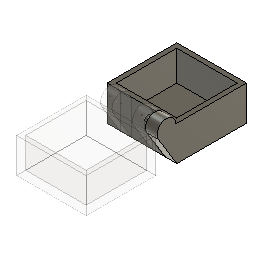
Day20BoxWithHinges (Autodesk Fusion 360 design; units mm, degrees)
part number: 2025-12-04-14-52-37-704
part number: 2025-12-04-18-52-37-317
part number: 2025-12-04-21-05-21-609
Autodesk Fusion 360 part; units mm, degrees
sketch "Sketch1" plane through (0, 0, 0) normal (0, 0, 1) x (1, 0, 0) in component "BoxBottom"
  line L0 (0, 0) -> (30, 0)
  line L1 (30, 0) -> (30, 30)
  line L2 (30, 30) -> (0, 30)
  line L3 (0, 30) -> (0, 0)
  dimension "d3" = 30
  dimension "d4" = 30
  constraint horizontal L0
  constraint vertical L1
  constraint horizontal L2
  constraint vertical L3
  constraint coincident L0.start L3.end
  measures "d3" distance of L0.start L2.end
  measures "d4" distance of L1.end L2.end
extrude "Extrude1" add sketch "Sketch1" along normal blind 15 makes body 1 in component "BoxBottom"
shell "Shell1" thickness 2 removed faces 1 at (10, 20, 15) on bodies 1 in component "BoxBottom"
sketch "Sketch1 (2)" plane through (0, 0, 0) normal (0, 0, 1) x (1, 0, 0) in component "BoxTop"
  line L0 (0, 0) -> (30, 0)
  line L1 (30, 0) -> (30, 30)
  line L2 (30, 30) -> (0, 30)
  line L3 (0, 30) -> (0, 0)
  dimension "d3_1" = 30
  dimension "d4_1" = 30
  constraint horizontal L0
  constraint vertical L1
  constraint horizontal L2
  constraint vertical L3
  constraint coincident L0.start L3.end
  measures "d3_1" distance of L0.start L2.end
  measures "d4_1" distance of L1.end L2.end
extrude "Extrude1'" add sketch "Sketch1 (2)" along normal blind 15 separate body makes body 2 in component "BoxTop"
shell "Shell1'" thickness 2 removed faces 1 at (10, 20, 15) on bodies 2 in component "BoxTop"
sketch "Sketch2" plane through (30, 0, 0) normal (1, 0, 0) x (0, 1, 0) in component "BoxBottom"
  line L0 (0, 0) -> (30, 0)
  line L1 (30, 0) -> (30, 15)
  line L2 (30, 15) -> (0, 15)
  line L3 (0, 15) -> (0, 0)
  line L4 (0, 15) -> (-4.5, 15)
  circle A0 centre (-4.5, 15) radius 4
  line L5 (0, 0) -> (-7.9106, 12.9101)
  dimension "d16" = 4.5
  dimension "d17" = 8
  constraint coincident L2.end L3.start
  constraint perpendicular L3 L4
  constraint coincident L4.end A0.centre
  constraint coincident L0.start L3.end
  constraint coincident A0 L5.end
  constraint tangent A0 L5
  measures "d16" distance of L2.end L4.end
  measures "d17" diameter of A0
extrude "Extrude2" add sketch "Sketch2" against normal blind 5 contours L3 L4 A0 L5 | A0 bodies 1 in component "BoxBottom"
sketch "Sketch3" plane through (25, 0, 0) normal (-1, 0, 0) x (0, -1, 0) in component "BoxBottom"
  line L0 (0.5, 15) -> (0, 15)
  line L1 (0, 15) -> (0, 0)
  line L2 (0, 0) -> (7.9106, 12.9101)
  arc A0 (7.9106, 12.9101) -> (0.5, 15) centre (4.5, 15) ccw
  circle A1 centre (4.5, 15) radius 2
  dimension "d20" = 4
  constraint concentric A0 A1
  measures "d20" diameter of A1
extrude "Extrude3" add sketch "Sketch3" along normal blind 3.8 draft -14 contours A1 bodies 1 in component "BoxBottom"
fillet "Fillet1" radius 1 1 edges at (21.2, -3.5187, 15.3806) on bodies 1 in component "BoxBottom"
sketch "Sketch2 (2)" plane through (5, 0, 0) normal (1, 0, 0) x (0, 1, 0) in component "BoxTop"
  circle A0 centre (-4.5, 15) radius 2
  line L0 (-8.5, 15) -> (-9, 15)
  line L1 (-9, 15) -> (-9, 0)
  line L2 (-9, 0) -> (-1.0894, 12.9101)
  arc A1 (-1.0894, 12.9101) -> (-8.5, 15) centre (-4.5, 15) ccw
  circle A2 centre (-4.5, 15) radius 0.2713
  arc A3 (-1.0894, 12.9101) -> (-8.5, 15) centre (-4.5, 15) ccw
  line L3 (-9, 0) -> (-1.0894, 12.9101)
  circle A4 centre (-4.5, 15) radius 4
  line L4 (0, 15) -> (-0.5, 15)
  line L5 (0, 15) -> (30, 15)
  line L6 (0, 0) -> (-7.9106, 12.9101)
  line L7 (0, 0) -> (0, 15)
  constraint concentric A3 A4
  constraint coincident L0.start A4
  constraint coincident A4 L4.end
  constraint horizontal L4
  constraint coincident L4.start L5
  constraint coincident L6.start L7.start
  constraint coincident A4 L6.end
  constraint tangent A4 L6
extrude "Extrude2'" add sketch "Sketch2 (2)" along normal blind 5 from surface at 0.6 separate body contours A0 | L0 L1 L2 L3 A4 L6 | A1 A3 A4 | L2 L3 A4 L6 makes body 3 in component "BoxTop"
ref_plane "WorkPlane1" through (15, 15, 7.5) normal (1, 0, 0) x (0, 1, 0) in component "BoxTop"
mirror "Mirror1" about plane through (15, 15, 7.5) normal (1, 0, 0) of bodies 3 makes body 4 in component "BoxTop"
component "BoxBottom" placed x (1, 0, 0) y (0, 1, 0) z (0, 0, 1) at (0, 0, 0)
component "BoxTop" placed x (-1, 0, 0) y (0, -1, 0) z (0, 0, 1) at (30, -9, 0)
equation "Box_Width = 30 mm"
equation "Box_Height = 15 mm"
equation "d3 = Box_Width"
equation "d4 = Box_Width"
equation "d5 = Box_Height"
equation "WallThickness = 2 mm"
equation "d3_1 = Box_Width"
equation "d4_1 = Box_Width"
equation "d5_1 = Box_Height"
equation "WallThickness_1 = 2 mm"
